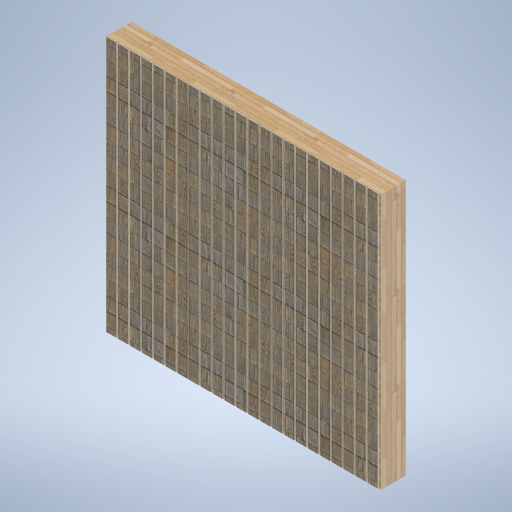
# Autodesk Inventor part: front_wall_block05
Saved by Autodesk Inventor 2024.2 (Build 282272000, 272)
## iProperties
Created: 2024-05-22
Part Number: front_wall_block05
Material: Wood (Maple)
Document SubType Name: Modeling
Designer: LOSTER_1
Density: 0.67 g/cm^3
Appearance: Natural Maple - Glossy Dark Tint
Author: LOSTER_1
Autodesk Inventor part; units mm, degrees
ref_plane "YZ Plane" through (0, 0, 0) normal (1, 0, 0) x (0, 1, 0)
ref_plane "XZ Plane" through (0, 0, 0) normal (0, 1, 0) x (-1, 0, 0)
ref_plane "XY Plane" through (0, 0, 0) normal (0, 0, 1) x (1, 0, 0)
sketch "Sketch2" plane through (0, 0, 0) normal (0, 0, 1) x (1, 0, 0)
  line L0 (-4421.0356, 1506.0734) -> (-1203.9241, 1506.0734)
  line L1 (-4421.0356, -1493.9266) -> (-4421.0356, 1506.0734)
  line L2 (-1203.9241, -1493.9266) -> (-1203.9241, 1506.0734)
  line L3 (-4421.0356, -1493.9266) -> (-1203.9241, -1493.9266)
  point P0 (0, 0)
  constraints: 8 end point, 1 horizontal
extrude "Extrusion1" add sketch "Sketch2" along normal blind 300
sketch "Sketch3" plane through (-4421.0356, 1506.0734, 0) normal (0, 1, 0) x (1, 0, 0)
  line L0 (0, 0) -> (0, -300) projected
  line L1 (3217.1114, -300) -> (0, -300) projected
  line L2 (3217.1114, 0) -> (3217.1114, -300) projected
  line L3 (0, -300) -> (120, -300)
  line L4 (120, -300) -> (120, -289.5168)
  line L5 (120, -289.5168) -> (139.7528, -289.5168)
  line L6 (139.7528, -289.5168) -> (139.7528, -300)
  line L7 (139.7528, -300) -> (259.7528, -300)
  line L8 (259.7528, -300) -> (259.7528, -289.5168)
  line L9 (259.7528, -289.5168) -> (279.4741, -289.5168)
  line L10 (279.4741, -289.5168) -> (279.4741, -300)
  line L11 (279.4741, -300) -> (399.4741, -300)
  line L12 (399.4741, -300) -> (399.4741, -289.5168)
  line L13 (399.4741, -289.5168) -> (419.1954, -289.5168)
  line L14 (419.1954, -289.5168) -> (419.1954, -300)
  line L15 (419.1954, -300) -> (539.1954, -300)
  line L16 (539.1954, -300) -> (539.1954, -289.5168)
  line L17 (539.1954, -289.5168) -> (558.9167, -289.5168)
  line L18 (558.9167, -289.5168) -> (558.9167, -300)
  line L19 (558.9167, -300) -> (678.9167, -300)
  line L20 (678.9167, -300) -> (678.9167, -289.5168)
  line L21 (678.9167, -289.5168) -> (698.638, -289.5168)
  line L22 (698.638, -289.5168) -> (698.638, -300)
  line L23 (698.638, -300) -> (818.638, -300)
  line L24 (818.638, -300) -> (818.638, -289.5168)
  line L25 (818.638, -289.5168) -> (838.78, -289.5168)
  line L26 (838.78, -289.5168) -> (838.78, -300)
  line L27 (838.78, -300) -> (958.78, -300)
  line L28 (958.78, -300) -> (958.78, -289.5168)
  line L29 (958.78, -289.5168) -> (968.4344, -289.5168)
  line L30 (968.4344, -289.5168) -> (968.4344, -300)
  line L31 (968.4344, -300) -> (1088.4344, -300)
  line L32 (1088.4344, -300) -> (1088.4344, -289.5168)
  line L33 (1088.4344, -289.5168) -> (1107.9538, -289.5168)
  line L34 (1107.9538, -289.5168) -> (1107.9538, -300)
  line L35 (1107.9538, -300) -> (1227.9538, -300)
  line L36 (1227.9538, -300) -> (1227.9538, -289.5168)
  line L37 (1227.9538, -289.5168) -> (1247.6343, -289.5168)
  line L38 (1247.6343, -289.5168) -> (1247.6343, -300)
  line L39 (1247.6343, -300) -> (1367.6343, -300)
  line L40 (1367.6343, -300) -> (1367.6343, -289.5168)
  line L41 (1367.6343, -289.5168) -> (1387.5005, -289.5168)
  line L42 (1387.5005, -289.5168) -> (1387.5005, -300)
  line L43 (1387.5005, -300) -> (1507.5005, -300)
  line L44 (1507.5005, -300) -> (1507.5005, -289.5168)
  line L45 (1507.5005, -289.5168) -> (1527.3666, -289.5168)
  line L46 (1527.3666, -289.5168) -> (1527.3666, -300)
  line L47 (1527.3666, -300) -> (1647.3666, -300)
  line L48 (1647.3666, -300) -> (1647.3666, -289.5168)
  line L49 (1647.3666, -289.5168) -> (1666.918, -289.5168)
  line L50 (1666.918, -289.5168) -> (1666.918, -300)
  line L51 (1666.918, -300) -> (1786.918, -300)
  line L52 (1786.918, -300) -> (1786.918, -289.5168)
  line L53 (1786.918, -289.5168) -> (1807.2385, -289.5168)
  line L54 (1807.2385, -289.5168) -> (1807.2385, -300)
  line L55 (1807.2385, -300) -> (1927.2385, -300)
  line L56 (1927.2385, -300) -> (1927.2385, -289.5168)
  line L57 (1927.2385, -289.5168) -> (1947.1441, -289.5168)
  line L58 (1947.1441, -289.5168) -> (1947.1441, -300)
  line L59 (1947.1441, -300) -> (2067.1441, -300)
  line L60 (2067.1441, -300) -> (2067.1441, -289.5168)
  line L61 (2067.1441, -289.5168) -> (2087.6299, -289.5168)
  line L62 (2087.6299, -289.5168) -> (2087.6299, -300)
  line L63 (2087.6299, -300) -> (2207.6299, -300)
  line L64 (2207.6299, -300) -> (2207.6299, -289.5168)
  line L65 (2207.6299, -289.5168) -> (2227.399, -289.5168)
  line L66 (2227.399, -289.5168) -> (2227.399, -300)
  line L67 (2227.399, -300) -> (2347.399, -300)
  line L68 (2347.399, -300) -> (2347.399, -289.5168)
  line L69 (2347.399, -289.5168) -> (2366.9939, -289.5168)
  line L70 (2366.9939, -289.5168) -> (2366.9939, -300)
  line L71 (2366.9939, -300) -> (2486.9939, -300)
  line L72 (2486.9939, -300) -> (2486.9939, -289.5168)
  line L73 (2486.9939, -289.5168) -> (2506.6686, -289.5168)
  line L74 (2506.6686, -289.5168) -> (2506.6686, -300)
  line L75 (2506.6686, -300) -> (2626.6686, -300)
  line L76 (2626.6686, -300) -> (2626.6686, -289.5168)
  line L77 (2626.6686, -289.5168) -> (2646.4797, -289.5168)
  line L78 (2646.4797, -289.5168) -> (2646.4797, -300)
  line L79 (2646.4797, -300) -> (2766.4797, -300)
  line L80 (2766.4797, -300) -> (2766.4797, -289.5168)
  line L81 (2766.4797, -289.5168) -> (2786.4453, -289.5168)
  line L82 (2786.4453, -289.5168) -> (2786.4453, -300)
  line L83 (2786.4453, -300) -> (2906.4453, -300)
  line L84 (2906.4453, -300) -> (2906.4453, -289.5168)
  line L85 (2906.4453, -289.5168) -> (2926.3963, -289.5168)
  line L86 (2926.3963, -289.5168) -> (2926.3963, -300)
  line L87 (2926.3963, -300) -> (3046.3963, -300)
  line L88 (3046.3963, -300) -> (3046.3963, -289.5168)
  line L89 (3046.3963, -289.5168) -> (3066.5174, -289.5168)
  line L90 (3066.5174, -289.5168) -> (3066.5174, -300)
  line L91 (3066.5174, -300) -> (3186.5174, -300)
  line L92 (3186.5174, -300) -> (3186.5174, -289.5168)
  line L93 (3186.5174, -289.5168) -> (3217.1114, -289.5168)
  line L94 (3217.1114, -289.5168) -> (3217.1114, -300)
  line L95 (3217.1114, -300) -> (120, -300)
  point P0 (4421.0356, 0)
  dimension "d2" = 120
  dimension "d3" = 90
  dimension "d4" = 120
  dimension "d5" = 120
  dimension "d6" = 120
  dimension "d7" = 120
  dimension "d8" = 120
  dimension "d9" = 120
  dimension "d10" = 120
  dimension "d11" = 120
  dimension "d12" = 120
  dimension "d13" = 120
  dimension "d14" = 120
  dimension "d15" = 120
  dimension "d16" = 120
  dimension "d17" = 120
  dimension "d18" = 120
  dimension "d19" = 120
  dimension "d20" = 120
  dimension "d21" = 120
  dimension "d22" = 120
  dimension "d23" = 120
  dimension "d24" = 120
  dimension "d25" = 120
  constraints: 186 end point, 36 point on line, 32 vertical, 17 perpendicular, 2 horizontal, 1 collinear, 46 other
  measures "d2" distance of L0.end L3.end
  measures "d3" angle of L4 L3
  measures "d4" distance of L6.end L7.end
  measures "d5" distance of L10.end L11.end
  measures "d6" distance of L14.end L15.end
  measures "d7" distance of L18.end L19.end
  measures "d8" distance of L22.end L23.end
  measures "d9" distance of L26.end L27.end
  measures "d10" distance of L30.end L31.end
  measures "d11" distance of L34.end L35.end
  measures "d12" distance of L38.end L39.end
  measures "d13" distance of L42.end L43.end
  measures "d14" distance of L46.end L47.end
  measures "d15" distance of L50.end L51.end
  measures "d16" distance of L54.end L55.end
  measures "d17" distance of L58.end L59.end
  measures "d18" distance of L62.end L63.end
  measures "d19" distance of L66.end L67.end
  measures "d20" distance of L70.end L71.end
  measures "d21" distance of L74.end L75.end
  measures "d22" distance of L78.end L79.end
  measures "d23" distance of L82.end L83.end
  measures "d24" distance of L86.end L87.end
  measures "d25" distance of L90.end L91.end
extrude "Extrusion2" cut sketch "Sketch3" against normal through all
body "Solid1"
